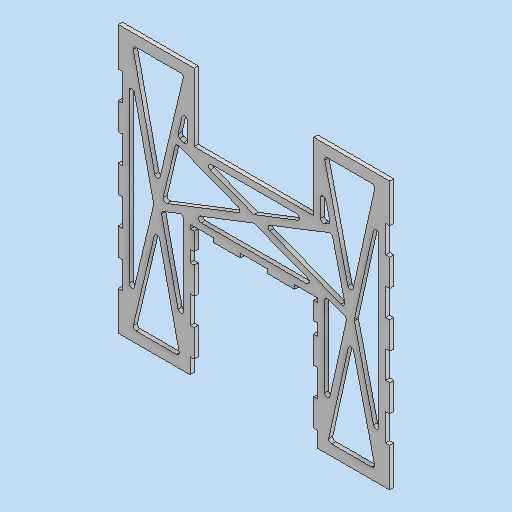
# Autodesk Inventor part: back plate
Saved by Autodesk Inventor 2026 (Build 300175000, 175)
## iProperties
Created: 2026-02-11
Part Number: back plate
Material: Generic
Document SubType Name: Modeling
Designer: mones
Density: 1 g/cm^3
Appearance: Default
Author: mones
Autodesk Inventor part; units mm, degrees
ref_plane "YZ Plane" through (0, 0, 0) normal (1, 0, 0) x (0, 1, 0)
ref_plane "XZ Plane" through (0, 0, 0) normal (0, 1, 0) x (-1, 0, 0)
ref_plane "XY Plane" through (0, 0, 0) normal (0, 0, 1) x (1, 0, 0)
sketch "Sketch1" plane through (0, 0, 0) normal (0, 0, 1) x (1, 0, 0)
  line L0 (-100, 98.5) -> (100, -98.5) construction
  line L1 (100, 98.5) -> (-100, -98.5) construction
  line L2 (-100, 98.5) -> (-100, 70)
  line L3 (-100, 50) -> (-100, 30)
  line L4 (-100, 10) -> (-100, -10)
  line L5 (-100, -30) -> (-100, -50)
  line L6 (-100, -70) -> (-100, -98.5)
  line L7 (-100, 98.5) -> (-100, 95.5)
  line L8 (-100, 98.5) -> (-100, 95.5)
  line L9 (-100, 98.5) -> (-97, 98.5)
  line L10 (-100, -70) -> (-97, -70)
  line L11 (-100, -50) -> (-97, -50)
  line L12 (-100, -30) -> (-97, -30)
  line L13 (-100, -10) -> (-97, -10)
  line L14 (-100, 10) -> (-97, 10)
  line L15 (-100, 30) -> (-97, 30)
  line L16 (-100, 50) -> (-97, 50)
  line L17 (-100, 70) -> (-97, 70)
  line L18 (-100, -98.5) -> (-100, -70)
  line L19 (-100, -50) -> (-100, -30)
  line L20 (-100, -10) -> (-100, 10)
  line L21 (-100, 30) -> (-100, 50)
  line L22 (-100, 70) -> (-100, 98.5)
  line L23 (100, 98.5) -> (97, 98.5)
  line L24 (100, -98.5) -> (100, -70)
  line L25 (100, -50) -> (100, -30)
  line L26 (100, -10) -> (100, 10)
  line L27 (100, 30) -> (100, 50)
  line L28 (100, 70) -> (97, 70)
  line L29 (100, 50) -> (97, 50)
  line L30 (100, 30) -> (97, 30)
  line L31 (100, 10) -> (97, 10)
  line L32 (100, -10) -> (97, -10)
  line L33 (100, -30) -> (97, -30)
  line L34 (100, -50) -> (97, -50)
  line L35 (100, -70) -> (97, -70)
  line L36 (100, -70) -> (100, -98.5)
  line L37 (100, -30) -> (100, -50)
  line L38 (100, 10) -> (100, -10)
  line L39 (100, 98.5) -> (100, 70)
  line L40 (100, 50) -> (100, 30)
  line L41 (-97, -98.5) -> (-47, -98.5)
  line L42 (-47, -98.5) -> (-100, -98.5)
  line L43 (-100, 98.5) -> (-47, 98.5)
  line L44 (100, -98.5) -> (47, -98.5)
  line L45 (47, -98.5) -> (47, -87)
  line L46 (47, -87) -> (47, -98.5)
  line L47 (100, -98.5) -> (47, -98.5)
  line L48 (47, 98.5) -> (97, 98.5)
  line L49 (47, 98.5) -> (100, 98.5)
  line L50 (-97, 98.5) -> (-47, 98.5)
  line L51 (-97, 70) -> (-97, 50)
  line L52 (-97, 30) -> (-97, 10)
  line L53 (-97, -10) -> (-97, -30)
  line L54 (-97, -50) -> (-97, -70)
  line L55 (97, -50) -> (97, -70)
  line L56 (97, -10) -> (97, -30)
  line L57 (97, 30) -> (97, 10)
  line L58 (97, 70) -> (97, 50)
  line L59 (-44, -68.5) -> (-44, -67)
  line L60 (-44, 71.5) -> (-44, 51.5)
  line L61 (-44, 48.5) -> (44, 48.5)
  line L62 (44, 51.5) -> (44, 71.5)
  line L63 (44, 71.5) -> (44, 98.5)
  line L64 (-44, 71.5) -> (-44, 98.5)
  line L65 (-44, 51.5) -> (-44, 48.5)
  line L66 (44, 51.5) -> (44, 48.5)
  line L67 (47, -98.5) -> (47, -87)
  line L68 (47, -87) -> (44, -87)
  line L69 (44, -87) -> (44, -67)
  line L70 (44, -67) -> (47, -67)
  line L71 (44, -47) -> (47, -47)
  line L72 (44, -27) -> (47, -27)
  line L73 (44, -18.5) -> (47, -18.5)
  line L74 (44, -87) -> (44, -67)
  line L75 (47, -67) -> (47, -47)
  line L76 (47, -27) -> (47, -18.5)
  line L77 (-44, -87) -> (-44, -68.5)
  line L78 (47, 98.5) -> (44, 98.5)
  line L79 (-44, 98.5) -> (-47, 98.5)
  line L80 (-47, -87) -> (-47, -98.5)
  line L81 (-47, -98.5) -> (-47, -87)
  line L82 (-47, -98.5) -> (-47, -87)
  line L83 (-47, -87) -> (-44, -87)
  line L84 (-44, -87) -> (-44, -67)
  line L85 (-44, -67) -> (-47, -67)
  line L86 (-44, -47) -> (-47, -47)
  line L87 (-44, -27) -> (-47, -27)
  line L88 (-44, -18.5) -> (-47, -18.5)
  line L89 (-44, -87) -> (-44, -67)
  line L90 (-47, -67) -> (-47, -47)
  line L91 (-47, -27) -> (-47, -18.5)
  line L92 (-47, -98.5) -> (-47, -87)
  line L93 (47, -67) -> (47, -47)
  line L94 (47, -47) -> (47, -47.4373)
  line L95 (44, -47) -> (44, -27)
  line L96 (44, -18.5) -> (44, -6.5)
  line L97 (-44, -18.5) -> (-44, -6.5)
  line L98 (-44, -47) -> (-44, -27)
  line L99 (47, -27) -> (47, -18.5)
  line L100 (-47, -27) -> (-47, -18.5)
  line L101 (-47, -98.5) -> (-47, -87)
  line L102 (-47, -67) -> (-47, -47)
  line L103 (-47, -5.5) -> (-47, -2.5)
  line L104 (-44, -6.5) -> (-44, -5.5)
  line L105 (-44, -5.5) -> (-47, -5.5)
  line L106 (44, -6.5) -> (44, -5.5)
  line L107 (44, -5.5) -> (47, -5.5)
  line L108 (47, -5.5) -> (47, -2.5)
  line L109 (-47, -2.5) -> (-30, -2.5)
  line L110 (-10, -2.5) -> (10, -2.5)
  line L111 (30, -2.5) -> (47, -2.5)
  line L112 (-30, -2.5) -> (-30, -5.5)
  line L113 (-10, -2.5) -> (-10, -5.5)
  line L114 (10, -2.5) -> (10, -5.5)
  line L115 (30, -2.5) -> (30, -5.5)
  line L116 (30, -5.5) -> (10, -5.5)
  line L117 (-10, -5.5) -> (-30, -5.5)
  line L118 (47, -2.5) -> (30, -2.5)
  line L119 (10, -2.5) -> (-10, -2.5)
  line L120 (-30, -2.5) -> (-47, -2.5)
  constraints: 242 end point, 84 perpendicular, 38 parallel, 10 vertical, 7 collinear, 7 horizontal, 4 point on line
extrude "Extrusion1" add sketch "Sketch1" along normal blind 3
sketch "Sketch3" plane through (0, 0, 3) normal (0, 0, 1) x (1, 0, 0)
  line L0 (-100, -70) -> (-100, -98.5) projected
  line L1 (-100, -98.5) -> (-47, -98.5) projected
  line L2 (-47, -98.5) -> (-47, -87) projected
  line L3 (-47, -87) -> (-44, -87) projected
  line L4 (-44, -87) -> (-44, -67) projected
  line L5 (-44, -67) -> (-47, -67) projected
  line L6 (-47, -67) -> (-47, -47) projected
  line L7 (-47, -47) -> (-44, -47) projected
  line L8 (-44, -47) -> (-44, -27) projected
  line L9 (-44, -27) -> (-47, -27) projected
  line L10 (-47, -27) -> (-47, -18.5) projected
  line L11 (-47, -18.5) -> (-44, -18.5) projected
  line L12 (-44, -18.5) -> (-44, -5.5) projected
  line L13 (-44, -5.5) -> (-47, -5.5) projected
  line L14 (-47, -5.5) -> (-47, -2.5) projected
  line L15 (-47, -2.5) -> (-30, -2.5) projected
  line L16 (-30, -2.5) -> (-30, -5.5) projected
  line L17 (-30, -5.5) -> (-10, -5.5) projected
  line L18 (-10, -5.5) -> (-10, -2.5) projected
  line L19 (-10, -2.5) -> (10, -2.5) projected
  line L20 (10, -2.5) -> (10, -5.5) projected
  line L21 (10, -5.5) -> (30, -5.5) projected
  line L22 (30, -5.5) -> (30, -2.5) projected
  line L23 (30, -2.5) -> (47, -2.5) projected
  line L24 (47, -2.5) -> (47, -5.5) projected
  line L25 (47, -5.5) -> (44, -5.5) projected
  line L26 (44, -5.5) -> (44, -18.5) projected
  line L27 (44, -18.5) -> (47, -18.5) projected
  line L28 (47, -18.5) -> (47, -27) projected
  line L29 (47, -27) -> (44, -27) projected
  line L30 (44, -27) -> (44, -47) projected
  line L31 (44, -47) -> (47, -47) projected
  line L32 (47, -47) -> (47, -67) projected
  line L33 (47, -67) -> (44, -67) projected
  line L34 (44, -67) -> (44, -87) projected
  line L35 (44, -87) -> (47, -87) projected
  line L36 (47, -87) -> (47, -98.5) projected
  line L37 (47, -98.5) -> (100, -98.5) projected
  line L38 (100, -98.5) -> (100, -70) projected
  line L39 (100, -70) -> (97, -70) projected
  line L40 (97, -70) -> (97, -50) projected
  line L41 (97, -50) -> (100, -50) projected
  line L42 (100, -50) -> (100, -30) projected
  line L43 (100, -30) -> (97, -30) projected
  line L44 (97, -30) -> (97, -10) projected
  line L45 (97, -10) -> (100, -10) projected
  line L46 (100, -10) -> (100, 10) projected
  line L47 (100, 10) -> (97, 10) projected
  line L48 (97, 10) -> (97, 30) projected
  line L49 (97, 30) -> (100, 30) projected
  line L50 (100, 30) -> (100, 50) projected
  line L51 (100, 50) -> (97, 50) projected
  line L52 (97, 50) -> (97, 70) projected
  line L53 (97, 70) -> (100, 70) projected
  line L54 (100, 70) -> (100, 98.5) projected
  line L55 (100, 98.5) -> (44, 98.5) projected
  line L56 (44, 98.5) -> (44, 48.5) projected
  line L57 (44, 48.5) -> (-44, 48.5) projected
  line L58 (-44, 48.5) -> (-44, 98.5) projected
  line L59 (-44, 98.5) -> (-100, 98.5) projected
  line L60 (-100, 98.5) -> (-100, 70) projected
  line L61 (-100, 70) -> (-97, 70) projected
  line L62 (-97, 70) -> (-97, 50) projected
  line L63 (-97, 50) -> (-100, 50) projected
  line L64 (-100, 50) -> (-100, 30) projected
  line L65 (-100, 30) -> (-97, 30) projected
  line L66 (-97, 30) -> (-97, 10) projected
  line L67 (-97, 10) -> (-100, 10) projected
  line L68 (-100, 10) -> (-100, -10) projected
  line L69 (-100, -10) -> (-97, -10) projected
  line L70 (-97, -10) -> (-97, -30) projected
  line L71 (-97, -30) -> (-100, -30) projected
  line L72 (-100, -30) -> (-100, -50) projected
  line L73 (-100, -50) -> (-97, -50) projected
  line L74 (-97, -50) -> (-97, -70) projected
  line L75 (-97, -70) -> (-100, -70) projected
  line L76 (100, 98.5) -> (100, -98.5)
  line L77 (100, -98.5) -> (52, -98.5)
  line L78 (-100, -98.5) -> (-100, 98.5)
  line L79 (92, -62.6123) -> (92, 60.5962)
  line L80 (44, 70) -> (44, 48.5)
  line L81 (44, 48.5) -> (-44, 48.5)
  line L82 (-44, 90.5) -> (-44, 98.5)
  line L83 (-31.4404, 43.5) -> (31.4404, 43.5)
  line L84 (-47, -2.5) -> (47, -2.5)
  line L85 (47, -2.5) -> (47, -98.5)
  line L86 (86.9494, 90.5) -> (54.1004, 90.5)
  line L87 (-54.1003, 90.5) -> (-86.9494, 90.5)
  line L88 (-49, 98.5) -> (-44, 98.5)
  line L89 (44, 98.5) -> (100, 98.5)
  line L90 (-49, 62.6123) -> (-49, 49.106)
  line L91 (-52, -1.3809) -> (-52, -60.5962)
  line L92 (-86.8996, -90.5) -> (-57.0506, -90.5)
  line L93 (57.0506, -90.5) -> (86.8996, -90.5)
  line L94 (-47, -87) -> (-47, -2.5)
  line L95 (48.1131, -96.5027) -> (94.4411, 89.9605) construction
  line L96 (89.5589, 91.0395) -> (52.9953, -97.5816) construction
  line L97 (91.1219, -97.62) -> (51.4323, 91.0778) construction
  line L98 (46.5677, 89.9222) -> (95.9865, -96.4643) construction
  line L99 (-48.0939, 45.83) -> (66.8796, -4.0853) construction
  line L100 (72.1832, -0.9411) -> (-49.9061, 41.17) construction
  line L101 (-72.1832, -0.9411) -> (49.9061, 41.17) construction
  line L102 (51.7965, 47.4375) -> (54.6694, 48.6847)
  line L103 (55.1886, 43.4634) -> (50.0836, 41.2471)
  line L104 (-55.3126, 43.2723) -> (-49.9061, 41.17)
  line L105 (-95.9865, -96.4643) -> (-46.5677, 89.9222) construction
  line L106 (-51.4322, 91.0779) -> (-91.1219, -97.62) construction
  line L107 (-92.9953, 83.4184) -> (-49.5589, -89.9605) construction
  line L108 (-54.4411, -91.0395) -> (-88.113, 84.4973) construction
  line L109 (-55.9529, -61.0278) -> (-68.0035, -6.4986)
  line L110 (-54.7249, 0.4831) -> (-66.7755, -4.203)
  line L111 (-73.3815, -22.9452) -> (-88.8455, -88.0377)
  line L112 (-73.0713, 16.4338) -> (-88.113, 84.4973)
  line L113 (-69.1726, 16.4031) -> (-52.1544, 88.0377)
  line L114 (-88.0423, -63.0248) -> (-73.9479, -3.697)
  line L115 (-88.0353, 60.9743) -> (-73.9408, -2.8032)
  line L116 (-69.4828, -22.9759) -> (-55.0977, -88.0684)
  line L117 (-69.7951, -9.977) -> (-69.7901, -10)
  line L118 (-77.699, -30.3026) -> (-77.6271, -30)
  line L119 (-88.9023, 88.0684) -> (-86.6673, 77.9551)
  line L120 (-91.5495, 76.8762) -> (-89.5589, 91.0395) construction
  line L121 (-94.4411, 89.9605) -> (-86.6673, 77.9551) construction
  line L122 (-91.9882, 60.5427) -> (-91.9882, -62.5626)
  line L123 (-49, 90.5) -> (-48.9998, 90.5)
  line L124 (-51.7248, 47.242) -> (-54.6622, 48.3842)
  line L125 (-58.6381, 49.9303) -> (-58.695, 49.9524)
  line L126 (-52.9458, 63.0746) -> (-55.8832, 50.7105)
  line L127 (-57.9833, 41.8706) -> (-66.8631, 4.4925)
  line L128 (-64.1924, 2.1662) -> (-11.6916, 22.5818)
  line L129 (0, 27.1282) -> (32.1652, 39.636)
  line L130 (-32.1652, 39.636) -> (0, 27.1282)
  line L131 (-11.6916, 26.3098) -> (-49.9061, 41.17)
  line L132 (48.0939, 45.83) -> (42.727, 43.5) construction
  line L133 (0, 24.9502) -> (-70.371, -5.6011) construction
  line L134 (49.8895, 41.1635) -> (11.6916, 26.3098)
  line L135 (-0.7248, 21.4816) -> (-39.6013, 6.364)
  line L136 (49, 49.272) -> (49, 62.6123)
  line L137 (55.8188, 50.9816) -> (52.9458, 63.0746)
  line L138 (38.8765, 2.5) -> (-38.8765, 2.5)
  line L139 (39.6013, 6.364) -> (0.7248, 21.4816)
  line L140 (66.8631, 4.4925) -> (57.9309, 42.0911)
  line L141 (55.9529, -61.0278) -> (68.036, -6.3515)
  line L142 (11.6916, 22.5818) -> (64.1924, 2.1662)
  line L143 (73.0714, 16.4337) -> (88.9023, 88.0684)
  line L144 (52.1545, 88.0377) -> (69.1727, 16.4031)
  line L145 (73.9479, -3.697) -> (88.0542, -63.0746)
  line L146 (67.4597, -4.469) -> (54.7248, 0.4831)
  line L147 (88.0471, 61.0278) -> (73.9408, -2.8032)
  line L148 (69.4828, -22.9759) -> (55.0977, -88.0684)
  line L149 (88.8455, -88.0377) -> (73.3815, -22.9452)
  line L150 (52, -60.5962) -> (52, -1.3809)
  arc A0 (-86.9494, 90.5) -> (-88.9023, 88.0684) centre (-86.9494, 88.5) ccw
  arc A1 (-52.1544, 88.0377) -> (-54.1003, 90.5) centre (-54.1003, 88.5) ccw
  arc A2 (-49, 62.6123) -> (-52.9458, 63.0746) centre (-51, 62.6123) ccw
  arc A3 (-55.8832, 50.7105) -> (-54.6622, 48.3842) centre (-53.9373, 50.2482) ccw
  arc A4 (-51.7248, 47.242) -> (-49, 49.106) centre (-51, 49.106) ccw
  arc A5 (-31.4404, 43.5) -> (-32.1652, 39.636) centre (-31.4404, 41.5) ccw
  arc A6 (32.1652, 39.636) -> (31.4404, 43.5) centre (31.4404, 41.5) ccw
  arc A7 (49, 49.272) -> (51.7965, 47.4375) centre (51, 49.272) ccw
  arc A8 (52.9458, 63.0746) -> (49, 62.6123) centre (51, 62.6123) ccw
  arc A9 (54.6694, 48.6847) -> (55.8188, 50.9816) centre (53.8729, 50.5193) ccw
  arc A10 (11.6916, 26.3098) -> (11.6916, 22.5818) centre (12.4164, 24.4458) ccw
  arc A11 (57.9309, 42.0911) -> (55.1886, 43.4634) centre (55.985, 41.6288) ccw
  arc A12 (64.1924, 2.1662) -> (66.8631, 4.4925) centre (64.9173, 4.0303) ccw
  arc A13 (69.1727, 16.4031) -> (73.0714, 16.4337) centre (71.1186, 16.8653) ccw
  arc A14 (88.9023, 88.0684) -> (86.9494, 90.5) centre (86.9494, 88.5) ccw
  arc A15 (54.1004, 90.5) -> (52.1545, 88.0377) centre (54.1004, 88.5) ccw
  arc A16 (92, 60.5962) -> (88.0471, 61.0278) centre (90, 60.5962) ccw
  arc A17 (73.9408, -2.8032) -> (73.9479, -3.697) centre (75.8937, -3.2347) ccw
  arc A18 (88.0542, -63.0746) -> (92, -62.6123) centre (90, -62.6123) ccw
  arc A19 (86.8996, -90.5) -> (88.8455, -88.0377) centre (86.8996, -88.5) ccw
  arc A20 (55.0977, -88.0684) -> (57.0506, -90.5) centre (57.0506, -88.5) ccw
  arc A21 (73.3815, -22.9452) -> (69.4828, -22.9759) centre (71.4357, -23.4075) ccw
  arc A22 (52, -60.5962) -> (55.9529, -61.0278) centre (54, -60.5962) ccw
  arc A23 (68.036, -6.3515) -> (67.4597, -4.469) centre (66.0832, -5.9199) ccw
  arc A24 (54.7248, 0.4831) -> (52, -1.3809) centre (54, -1.3809) ccw
  arc A25 (38.8765, 2.5) -> (39.6013, 6.364) centre (38.8765, 4.5) ccw
  arc A26 (0.7248, 21.4816) -> (-0.7248, 21.4816) centre (0, 19.6176) ccw
  arc A27 (-39.6013, 6.364) -> (-38.8765, 2.5) centre (-38.8765, 4.5) ccw
  arc A28 (-11.6916, 22.5818) -> (-11.6916, 26.3098) centre (-12.4164, 24.4458) ccw
  arc A29 (-55.3126, 43.2723) -> (-57.9833, 41.8706) centre (-56.0374, 41.4083) ccw
  arc A30 (-66.8631, 4.4925) -> (-64.1924, 2.1662) centre (-64.9173, 4.0303) ccw
  arc A31 (-73.0713, 16.4338) -> (-69.1726, 16.4031) centre (-71.1185, 16.8653) ccw
  arc A32 (-88.0353, 60.9743) -> (-91.9882, 60.5427) centre (-89.9882, 60.5427) ccw
  arc A33 (-73.9479, -3.697) -> (-73.9408, -2.8032) centre (-75.8937, -3.2347) ccw
  arc A34 (-91.9882, -62.5626) -> (-88.0423, -63.0248) centre (-89.9882, -62.5626) ccw
  arc A35 (-66.7755, -4.203) -> (-68.0035, -6.4986) centre (-66.0507, -6.067) ccw
  arc A36 (-52, -1.3809) -> (-54.7249, 0.4831) centre (-54, -1.3809) ccw
  arc A37 (-55.9529, -61.0278) -> (-52, -60.5962) centre (-54, -60.5962) ccw
  arc A38 (-57.0506, -90.5) -> (-55.0977, -88.0684) centre (-57.0506, -88.5) ccw
  arc A39 (-88.8455, -88.0377) -> (-86.8996, -90.5) centre (-86.8996, -88.5) ccw
  arc A40 (-69.4828, -22.9759) -> (-73.3815, -22.9452) centre (-71.4357, -23.4075) ccw
  line L151 (-86.9494, 90.5) -> (-54.1003, 90.5)
  line L152 (-71.1885, 7.9138) -> (-71.1885, 7.9135)
  line L153 (-74.6801, 23.7132) -> (-73.0713, 16.4338)
  line L154 (-81.7299, 90.5) -> (-86.9494, 90.5)
  line L155 (-89.4396, 90.5) -> (-89.4397, 90.5)
  line L156 (-88.113, 84.4973) -> (-88.9068, 88.089)
  line L157 (50.0836, 41.2471) -> (49.8895, 41.1635)
  point P0 (51.5538, 90.5)
  point P1 (-11.1386, 20.1145)
  point P2 (-89.6243, -90.5)
  point P3 (-54.5446, -90.5)
  point P4 (-52, -80.2167)
  point P5 (89.4543, 90.5)
  dimension "d86" = 2
  dimension "d87" = 2
  dimension "d88" = 2
  dimension "d89" = 2
  dimension "d90" = 2
  constraints: 166 end point, 83 point on circle, 82 tangent, 51 parallel, 41 centre point, 36 equal radius, 25 point on line, 8 perpendicular, 3 horizontal, 1 collinear, 1 midpoint
  measures "d86" radius of A0
  measures "d87" radius of A10
  measures "d88" radius of A29
  measures "d89" radius of A34
  measures "d90" radius of A35
extrude "Extrusion2" cut sketch "Sketch3" against normal blind 3 contours A18 L145 A17 L147 A16 L79 | L83 A6 L129 L130 A5 | A14 L143 A13 L144 A15 L86 | A1 L113 A31 L112 L119 A0 L87 | L90 A4 L124 A3 L126 A2 | L91 A37 L109 A35 L110 A36 | A39 L111 A40 L116 A38 L92 | A20 L148 A21 L149 A19 L93 | A7 L136 A8 L137 A9 L102 | A11 L140 A12 L142 A10 L134 L157 L103 | L104 L131 A28 L128 A30 L127 A29 | A34 L122 A32 L115 A33 L114 | A26 L139 A25 L138 A27 L135 | A22 L150 A24 L146 A23 L141
body "Solid1"
